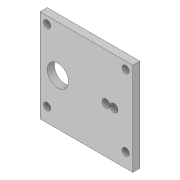
# Autodesk Inventor part: PARTIMP
Saved by Autodesk Inventor 2019 (Build 230136000, 136)
## iProperties
Created: 2019-10-08
Part Number: PARTIMP
Material: Generic
Document SubType Name: Modeling
Designer: Admin
Density: 1 g/cm^3
Appearance: Default
Author: Admin
Autodesk Inventor part; units mm, degrees
ref_plane "YZ Plane" through (0, 0, 0) normal (1, 0, 0) x (0, 1, 0)
ref_plane "XZ Plane" through (0, 0, 0) normal (0, 1, 0) x (-1, 0, 0)
ref_plane "XY Plane" through (0, 0, 0) normal (0, 0, 1) x (1, 0, 0)
sketch "Sketch1" plane through (0, 0, 0) normal (0, 0, 1) x (1, 0, 0)
  line L0 (0, 0) -> (130, 0)
  line L1 (130, 0) -> (130, 130)
  line L2 (130, 130) -> (0, 130)
  line L3 (0, 130) -> (0, 0)
  dimension "d0" = 130
  dimension "d1" = 130
  constraints: 8 end point, 2 parallel, 1 horizontal, 1 perpendicular
  measures "d0" distance of L2.end L1.end
  measures "d1" distance of L1.end L0.end
extrude "Extrusion1" add sketch "Sketch1" along normal blind 10
sketch "Sketch2" plane through (0, 0, 10) normal (0, 0, 1) x (1, 0, 0)
  line L0 (130, 130) -> (0, 130) projected
  line L1 (0, 130) -> (10, 130)
  line L2 (10, 130) -> (10, 20)
  line L3 (0, 0) -> (130, 0) projected
  line L4 (10, 20) -> (120, 20)
  line L5 (120, 20) -> (120, 130)
  line L6 (120, 130) -> (120, 10)
  line L7 (120, 10) -> (10, 10)
  line L8 (10, 10) -> (10, 120)
  arc A0 (10, 130) -> (10, 123.825) centre (10, 126.9125) ccw
  line L9 (120, 130) -> (120, 120)
  circle A1 centre (120, 120) radius 5
  circle A2 centre (10, 120) radius 5
  circle A3 centre (10, 20) radius 5
  circle A4 centre (120, 20) radius 5
  dimension "d4" = 10
  dimension "d5" = 110
  dimension "d6" = 110
  dimension "d7" = 110
  dimension "d8" = 120
  dimension "d9" = 110
  dimension "d10" = 110
  dimension "d11" = 10
  dimension "d12" = 10
  dimension "d13" = 10
  dimension "d14" = 10
  dimension "d15" = 10
  constraints: 16 end point, 6 point on line, 5 centre point, 4 coincident, 2 perpendicular, 2 point on circle, 1 tangent
  measures "d4" distance of L0.end L1.end
  measures "d5" distance of L1.end L2.end
  measures "d6" distance of L2.end L4.end
  measures "d7" distance of L4.end L5.end
  measures "d8" distance of L5.end L6.end
  measures "d9" distance of L6.end L7.end
  measures "d10" distance of L7.end L8.end
  measures "d11" distance of L5.end L9.end
  measures "d12" diameter of A1
  measures "d13" diameter of A2
  measures "d14" diameter of A3
  measures "d15" diameter of A4
extrude "Extrusion2" cut sketch "Sketch2" against normal blind 10 contours A1 L5 | L5 A1 | A2 L2 | L2 A0 A2 | A0 L2 A2 | A4 L6 L5 | L5 L4 A4 | A3 L4 L2 | L2 L8 A3 | L6 A4 L4 | L4 A3 L8 picked at (9.758, 124.2455) picked at (8.4412, 122.3255)
sketch "Sketch3" plane through (0, 0, 10) normal (0, 0, 1) x (1, 0, 0)
  line L0 (130, 0) -> (130, 130) projected
  line L1 (130, 0) -> (130, 65)
  line L2 (130, 65) -> (92.5, 65)
  circle A0 centre (92.5, 65) radius 5.5
  point P0 (0, 0)
  dimension "d18" = 65
  dimension "d19" = 37.5
  dimension "d20" = 11
  constraints: 4 end point, 1 centre point, 1 coincident, 1 midpoint, 1 perpendicular
  measures "d18" distance of L0.start L1.end
  measures "d19" distance of L1.end L2.end
  measures "d20" diameter of A0
extrude "Extrusion3" cut sketch "Sketch3" against normal through all
sketch "Sketch4" plane through (0, 0, 0) normal (0, 0, -1) x (-1, 0, 0)
  line L0 (0, 130) -> (0, 0) projected
  line L1 (0, 130) -> (0, 65)
  line L2 (0, 65) -> (-25, 65)
  circle A0 centre (-25, 65) radius 15
  dimension "d23" = 65
  dimension "d24" = 25
  dimension "d25" = 30
  constraints: 4 end point, 1 centre point, 1 coincident, 1 midpoint, 1 perpendicular
  measures "d23" distance of L0.start L1.end
  measures "d24" distance of L1.end L2.end
  measures "d25" diameter of A0
extrude "Extrusion4" cut sketch "Sketch4" against normal blind 10
sketch "Sketch5" plane through (0, 0, 0) normal (0, 0, -1) x (-1, 0, 0)
  line L0 (-128.5875, 65.0875) -> (-103.5875, 65.0875)
  circle A0 centre (-103.5875, 65.0875) radius 5.5
  point P0 (0, 0)
  dimension "d28" = 25
  dimension "d29" = 11
  constraints: 2 end point, 1 centre point, 1 coincident, 1 horizontal, 1 point on line
  measures "d28" distance of L0.start L0.end
  measures "d29" diameter of A0
extrude "Extrusion5" cut sketch "Sketch5" against normal blind 11
equation "\"d30\" = d29"
body "Solid1"
